Autodesk Fusion 360 part; units mm, degrees
(part 2 of 6)
  constraint perpendicular L499 L505
  constraint perpendicular L506 L507
  constraint perpendicular L505 L506
  constraint perpendicular L478 L508
  constraint parallel L412 L509
  constraint perpendicular L508 L510
  constraint horizontal L511
  constraint vertical L512
  constraint horizontal L513
  constraint vertical L514
  constraint coincident L510 L515.start
  constraint perpendicular L510 L515
  constraint coincident L509 L516.end
  constraint perpendicular L515 L516
  constraint coincident L515.end L516.start
  constraint tangent L509 A143
  constraint tangent L481 A144
  constraint tangent L410 A144
  constraint tangent L407 A145
  constraint tangent L403 A145
  constraint coincident L512.end L513.start
  constraint tangent L480 A147
  constraint tangent L481 A147
  constraint coincident L480 L517.start
  constraint perpendicular L412 L517
  constraint tangent A147 L517
  constraint coincident L481 L518.start
  constraint perpendicular L404 L518
  constraint tangent A147 L518
  constraint coincident L481 L519.start
  constraint perpendicular L481 L519
  constraint tangent A144 L519
  constraint perpendicular L519 L520
  constraint tangent A144 L520
  constraint coincident L410 L520.end
  constraint coincident L477 L521.start
  constraint perpendicular L477 L521
  constraint perpendicular L521 L522
  constraint tangent A145 L521
  constraint tangent A145 L522
  constraint coincident L407 L522.end
  constraint coincident L510 L523.start
  constraint perpendicular L510 L523
  constraint perpendicular L523 L524
  constraint tangent A143 L524
  constraint tangent A143 L523
  constraint coincident L509 L524.end
  constraint coincident L508 L525.start
  constraint perpendicular L508 L525
  constraint coincident L510 L526.end
  constraint perpendicular L510 L526
  constraint tangent A146 L525
  constraint tangent A146 L526
  constraint perpendicular L502 L527
  constraint perpendicular L527 L528
  constraint perpendicular L505 L529
  constraint perpendicular L529 L530
  constraint perpendicular L506 L531
  constraint perpendicular L531 L532
  constraint horizontal L533
  constraint vertical L534
  constraint horizontal L535
  constraint vertical L536
  constraint coincident L495 L534.end
  constraint parallel L504 L535
  constraint coincident L536 A148.centre
  constraint tangent L535 A148
  constraint tangent L535 A149
  constraint tangent L534 A149
  constraint coincident L506 A150.centre
  constraint tangent L507 A150
  constraint coincident L505 A151.centre
  constraint tangent L506 A151
  constraint coincident L501 A152.centre
  constraint tangent L502 A152
  constraint coincident L528.end A153.centre
  constraint coincident L530.end A154.centre
  constraint coincident L532.end A155.centre
  constraint coincident L497.end A156.centre
  constraint coincident L535 L537.start
  constraint perpendicular L535 L537
  constraint coincident L537.end A157.centre
  constraint perpendicular L536 L538
  constraint perpendicular L538 L539
  constraint coincident L539.end A158.centre
  constraint coincident A158 L540.end
  constraint tangent A158 L540
  constraint coincident A158 L541.start
  constraint coincident L503 L541.end
  constraint tangent A158 L541
  constraint perpendicular L503 L541
  constraint coincident A157 L542.end
  constraint tangent A157 L542
  constraint perpendicular L537 L543
  constraint coincident A157 L544.end
  constraint tangent A157 L544
  constraint coincident A156 L545.end
  constraint tangent A156 L545
  constraint perpendicular L497 L546
  constraint coincident A156 L547.end
  constraint tangent A156 L547
  constraint coincident A153 L548.end
  constraint tangent A153 L548
  constraint coincident L506 L549.end
  constraint perpendicular L506 L549
  constraint perpendicular L549 L550
  constraint perpendicular L549 L551
  constraint coincident A155 L552.end
  constraint tangent A155 L552
  constraint coincident A155 L553.end
  constraint tangent A155 L553
  constraint coincident A154 L554.end
  constraint tangent A154 L554
  constraint coincident L505 L555.end
  constraint perpendicular L505 L555
  constraint perpendicular L555 L556
  constraint coincident A154 L557.end
  constraint tangent A154 L557
  constraint coincident L502 L558.end
  constraint perpendicular L502 L558
  constraint perpendicular L558 L559
  constraint coincident A153 L560.end
  constraint tangent A153 L560
  constraint coincident A113.centre L561.start
  constraint coincident L403 L561.end
  constraint perpendicular L477 L561
  constraint coincident L410 L562.start
  constraint vertical L562
  constraint coincident A147.centre L563.end
  constraint parallel L563 L564
  constraint coincident L562.end L564.end
  constraint coincident A60.centre A139.centre
  constraint coincident L562 L565.end
  constraint perpendicular L562 L565
  constraint parallel L565 L566
  constraint perpendicular L566 L567
  constraint perpendicular L566 L568
  constraint coincident L562 L569.start
  constraint coincident L562 L570.end
  constraint perpendicular L520 L574
  constraint horizontal L575
  constraint vertical L576
  constraint horizontal L577
  constraint vertical L578
  constraint perpendicular L575 L579
  constraint coincident L573 L580.start
  constraint perpendicular L579 L581
  constraint perpendicular L573 L580
  constraint parallel L572 L580
  constraint coincident L562 L582.end
  constraint perpendicular L562 L582
  constraint midpoint L49 L583.start
  constraint coincident L580 L583.end
  constraint perpendicular L580 L583
  constraint coincident A51.centre A141.centre
  constraint perpendicular L562 L584
  constraint perpendicular L584 L585
  constraint coincident L507 L586.start
  constraint coincident L507 L586.end
  constraint perpendicular L586 L587
  constraint coincident L564 L588.end
  constraint perpendicular L584 L588
  constraint coincident A125.centre L589.start
  constraint perpendicular L500 L589
  constraint perpendicular L481 L590
  constraint coincident L404 L591.end
  constraint coincident L404 L592.end
  constraint parallel L404 L592
  constraint perpendicular L585 L593
  constraint coincident A57.centre A140.centre
  constraint perpendicular L593 L596
  constraint perpendicular L590 L595
  constraint coincident L562 L597.end
  constraint perpendicular L562 L597
  constraint coincident L562 L599.end
  constraint perpendicular L562 L599
  constraint coincident L404 L600.end
  constraint coincident L481 L601.end
  constraint parallel L590 L600
  constraint parallel L593 L601
  constraint perpendicular L566 L602
  constraint perpendicular L565 L603
  constraint coincident L571 L604.end
  constraint coincident L562 L609.start
  constraint perpendicular L602 L609
  constraint perpendicular L602 L608
  constraint perpendicular L607 L608
  constraint perpendicular L605 L606
  constraint perpendicular L603 L604
  constraint perpendicular L603 L605
  measures "d1" distance of L0.start L0.end
  measures "d2" distance of L12.start L485.end
  measures "d3" distance of L12.start L487.end
  measures "d4" distance of L10.start L489.end
  measures "d5" distance of L10.start L491.end
  measures "d6" distance of L486.end L496.end
  measures "d7" distance of L496.end L497.end
  measures "d8" distance of L490.end L498.end
  measures "d10" distance of L499.start L499.end
  measures "d11" distance of L500.start L500.end
  measures "d12" distance of L502 L503
  measures "d13" distance of L501 L506
  measures "d14" distance of L406 L506
  measures "d15" distance of L403 L404
  measures "d16" distance of L406.start L407.end
  measures "d17" distance of L406.start L508.end
  measures "d18" distance of L508.end L511.end
  measures "d19" distance of L508.end L513.end
  measures "d20" distance of L515.start L515.end
  measures "d22" diameter of A143
  measures "d23" diameter of A144
  measures "d24" diameter of A145
  measures "d25" diameter of A146
  measures "d26" diameter of A147
  measures "d27" distance of L501.end L527.end
  measures "d28" distance of L527.end L528.end
  measures "d29" distance of L505.end L529.end
  measures "d30" distance of L529.end L530.end
  measures "d31" distance of L506.end L531.end
  measures "d32" distance of L531.end L532.end
  measures "d33" distance of L533 L535
  measures "d34" diameter of A148
  measures "d35" diameter of A149
  measures "d36" diameter of A150
  measures "d37" diameter of A151
  measures "d38" diameter of A152
  measures "d39" diameter of A153
  measures "d40" diameter of A154
  measures "d41" diameter of A155
  measures "d42" diameter of A156
  measures "d43" distance of L537.start L537.end
  measures "d44" distance of L534.end L537
  measures "d45" diameter of A157
  measures "d46" distance of L535.end L538.end
  measures "d47" distance of L538.end L539.end
  measures "d48" diameter of A158
  measures "d49" distance of L537.start L543.end
  measures "d50" distance of L496.end L546.end
  measures "d51" distance of L549.end L550.end
  measures "d52" distance of L549.end L551.end
  measures "d53" distance of L555.end L556.end
  measures "d54" distance of L558.end L559.end
  measures "d55" distance of A113.centre L561.end
  measures "d56" distance of A112.centre A113.centre
  measures "d57" distance of L404 L562
  measures "d58" distance of A60.centre L565.end
  measures "d59" distance of A60.centre L566.end
  measures "d60" distance of L566.end L567.end
  measures "d61" distance of L566.end L568.end
  measures "d62" distance of L565.end L570.end
  measures "d63" distance of L565.end L569.start
  measures "d70" angle of L410 L574
  measures "d72" distance of L575.start L575.end
  measures "d73" distance of L575.start L577.end
  measures "d74" distance of A114.centre L575
  measures "d75" distance of A114.centre L576
  measures "d76" distance of L562 L576
  measures "d77" distance of L575.end L579.end
  measures "d80" distance of L583.start L583.end
  measures "d81" distance of A51.centre L562
  measures "d82" distance of A51.centre L584.end
  measures "d84" distance of L586.start L586.end
  measures "d87" distance of A125.centre L589.end
  measures "d88" angle of L562 L598
  measures "d89" angle of L591 L595
  measures "d90" angle of L594 L596
  measures "d91" distance of L590.end A57.centre
  measures "d92" distance of L593.end A57.centre
  measures "d93" distance of A60.centre L603.end
  measures "d94" distance of A60.centre L602.end
sketch "Sketch2" plane through (0, 0, 0) normal (0, 1, 0) x (1, 0, 0)
  line L0 (123.6133, -112.6772) -> (84.9842, -117.4397)
  line L1 (123.6486, -112.6772) -> (118.0197, -90.1409)
  line L2 (121.9175, -105.7465) -> (132.0216, -103.2228)
  line L3 (132.0216, -103.2228) -> (140.1031, -103.2228)
  line L4 (140.1031, -103.2228) -> (142.7339, -103.2228)
  line L5 (142.7339, -107.9103) -> (142.7339, -30.6526)
  line L6 (142.7339, -80.8214) -> (146.7556, -80.8214)
  line L7 (150.7772, -80.8214) -> (146.7556, -80.8214)
  line L8 (149.7839, -80.9328) -> (143.7839, -80.9328)
  circle A0 centre (149.7839, -83.4328) radius 2.5
  line L9 (143.7839, -89.4328) -> (150.9524, -85.6429)
  circle A1 centre (143.7839, -87.4328) radius 2
  line L10 (143.7839, -89.4328) -> (143.7839, -81.4328)
  line L11 (143.7839, -48.2006) -> (143.7839, -81.4328)
  line L12 (150.7772, -76.7997) -> (150.7772, -78.8106)
  line L13 (150.7772, -78.8106) -> (150.7772, -80.8214)
  line L14 (150.7772, -76.7997) -> (150.7772, -74.7889)
  line L15 (150.7772, -72.7781) -> (150.7772, -74.7889)
  line L16 (146.7556, -72.7781) -> (150.7772, -72.7781)
  line L17 (146.7556, -72.7781) -> (142.7339, -72.7781)
  line L18 (144.7094, -48.4919) -> (142.7339, -48.4919)
  line L19 (144.7094, -48.4919) -> (157.6917, -48.4919)
  line L20 (157.6917, -48.4919) -> (161.7839, -48.4919)
  line L21 (157.6917, -40.3375) -> (161.7839, -40.3375)
  line L22 (161.7839, -30.1978) -> (161.7839, -98.4956)
  line L23 (150.7772, -40.3375) -> (157.6917, -40.3375)
  line L24 (150.7772, -37.8883) -> (150.7772, -40.3375)
  line L25 (150.7772, -37.8883) -> (150.7772, -28.4944)
  circle A2 centre (155.7839, -27.151) radius 6
  line L26 (161.7839, -33.151) -> (153.5462, -33.151)
  line L27 (161.7839, -25.5411) -> (161.7839, -103.1522)
  line L28 (161.7839, -25.5411) -> (155.7839, -27.151)
  line L29 (155.7839, -27.151) -> (142.7339, -30.6526)
  line L30 (157.9757, -18.9558) -> (147.6976, -24.893)
  line L31 (143.7839, -15.9328) -> (143.7839, -48.2006)
  circle A3 centre (141.7839, -15.9328) radius 2
  line L32 (27.2428, -15.9328) -> (143.7839, -15.9328)
  line L33 (125.7839, -15.9328) -> (121.994, -8.7643)
  circle A4 centre (119.7839, -9.9328) radius 2.5
  line L34 (113.7839, -15.9328) -> (117.5738, -8.7643)
  line L35 (142.6281, 7.5847) -> (161.7839, -25.5411)
  line L36 (142.6281, 7.5847) -> (103.8578, -14.9931)
  line L37 (9.2428, -14.9931) -> (103.8578, -14.9931)
  circle A5 centre (27.2428, -17.9328) radius 2
  line L38 (27.2428, -15.9328) -> (20.0743, -19.7226)
  circle A6 centre (21.2428, -21.9328) radius 2.5
  line L39 (27.2428, -27.9328) -> (20.0743, -24.1429)
  line L40 (27.2428, -51.1815) -> (27.2428, -15.9328)
  line L41 (27.2428, -81.4328) -> (27.2428, -51.1815)
  line L42 (27.2428, -69.4328) -> (20.0743, -73.2226)
  circle A7 centre (21.2428, -75.4328) radius 2.5
  line L43 (27.2428, -81.4328) -> (20.0743, -77.6429)
  circle A8 centre (29.2428, -81.4328) radius 2
  line L44 (57.5469, -81.4328) -> (27.2428, -81.4328)
  line L45 (51.5469, -81.4328) -> (55.3368, -88.6012)
  circle A9 centre (57.5469, -87.4328) radius 2.5
  line L46 (63.5469, -81.4328) -> (59.7571, -88.6012)
  line L47 (63.5469, -81.6328) -> (63.5469, -117.0186)
  line L48 (63.5469, -81.4328) -> (57.5469, -81.4328)
  line L49 (63.5469, -81.6328) -> (63.5469, -81.4328)
  line L50 (63.5469, -81.4328) -> (63.7469, -81.4328)
  line L51 (63.7469, -81.4328) -> (86.36, -81.4328)
  line L52 (86.56, -81.4328) -> (86.36, -81.4328)
  line L53 (86.56, -81.4328) -> (86.56, -89.4328)
  line L54 (143.7839, -81.4328) -> (86.56, -81.4328)
  line L55 (98.56, -89.4328) -> (94.7701, -96.6012)
  circle A10 centre (92.56, -95.4328) radius 2.5
  line L56 (86.56, -89.4328) -> (90.3499, -96.6012)
  circle A11 centre (88.56, -87.4328) radius 2
  line L57 (86.56, -89.4328) -> (143.7839, -89.4328)
  line L58 (149.7839, -92.4665) -> (149.7839, -106.1494)
  line L59 (161.7839, -92.4665) -> (149.7839, -92.4665)
  circle A12 centre (155.7839, -98.4665) radius 6
  line L60 (161.7839, -103.1522) -> (123.6486, -112.6772)
  line L61 (84.9842, -117.4397) -> (66.9572, -117.4397)
  line L62 (9.2428, -110.3136) -> (66.9572, -117.4397)
  line L63 (21.2428, -99.0089) -> (21.2428, -111.7953)
  line L64 (9.2428, -99.0089) -> (21.2428, -99.0089)
  circle A13 centre (15.2428, -105.0089) radius 6
  line L65 (9.2428, -105.6569) -> (9.2428, -19.6497)
  line L66 (9.2428, -110.3136) -> (9.2428, -14.9931)
  line L67 (142.6281, 7.5847) -> (100.6075, 80.3275)
  line L68 (9.2428, -14.9931) -> (9.2428, 80.3275)
  line L69 (21.2428, 68.3275) -> (21.2428, 80.3275)
  line L70 (9.2428, 68.3275) -> (21.2428, 68.3275)
  circle A14 centre (15.2428, 74.3275) radius 6
  line L71 (91.1443, 80.3275) -> (91.1443, 68.3275)
  line L72 (91.1443, 68.3275) -> (107.5394, 68.3275)
  circle A15 centre (97.1443, 74.3275) radius 6
  line L73 (9.2428, 80.3275) -> (100.6075, 80.3275)
  line L74 (155.7839, -27.151) -> (97.1443, 74.3275)
  line L75 (15.2428, -105.0089) -> (15.2428, 74.3275)
  line L76 (21.2428, -21.9328) -> (15.2428, -21.9328)
  circle A16 centre (15.2428, 26.1974) radius 2.5
  circle A17 centre (126.4641, 23.5882) radius 2.5
  line L77 (15.2428, 68.3275) -> (9.2428, 68.3275)
  line L78 (21.2428, 80.3275) -> (21.2428, 74.3275)
  line L79 (9.2428, 68.3275) -> (9.2428, 80.3275)
  line L80 (21.2428, 80.3275) -> (9.2428, 80.3275)
  line L81 (21.2428, 80.3275) -> (91.1443, 80.3275)
  line L82 (91.1443, 80.3275) -> (91.1443, 74.3275)
  line L83 (107.5394, 68.3275) -> (97.1443, 68.3275)
  arc A18 (91.1443, 74.3275) -> (97.1443, 68.3275) centre (97.1443, 74.3275) ccw
  line L84 (91.1443, 80.3275) -> (100.6075, 80.3275)
  line L85 (100.6075, 80.3275) -> (142.6281, 7.5847)
  line L86 (142.6281, 7.5847) -> (103.8578, -14.9931)
  line L87 (103.8578, -14.9931) -> (9.2428, -14.9931)
  line L88 (9.2428, -110.3136) -> (9.2428, 68.3275)
  line L89 (9.2428, -99.0089) -> (15.2428, -99.0089)
  arc A19 (21.2428, -105.0089) -> (15.2428, -99.0089) centre (15.2428, -105.0089) ccw
  line L90 (21.2428, -105.0089) -> (21.2428, -111.7953)
  line L91 (9.2428, -110.3136) -> (21.2428, -111.7953)
  line L92 (21.2428, -111.7953) -> (66.9572, -117.4397)
  line L93 (66.9572, -117.4397) -> (84.9842, -117.4397)
  line L94 (63.5469, -117.0186) -> (63.5469, -81.4328)
  line L95 (63.5469, -81.4328) -> (59.7571, -88.6012)
  line L96 (63.5469, -81.4328) -> (51.5469, -81.4328)
  line L97 (55.3368, -88.6012) -> (51.5469, -81.4328)
  arc A20 (55.3368, -88.6012) -> (59.7571, -88.6012) centre (57.5469, -87.4328) ccw
  line L98 (51.5469, -81.4328) -> (27.2428, -81.4328)
  arc A21 (27.2428, -81.4328) -> (31.2428, -81.4328) centre (29.2428, -81.4328) ccw
  arc A22 (20.0743, -73.2226) -> (20.0743, -77.6429) centre (21.2428, -75.4328) ccw
  line L99 (27.2428, -81.4328) -> (20.0743, -77.6429)
  line L100 (20.0743, -73.2226) -> (27.2428, -69.4328)
  line L101 (27.2428, -81.4328) -> (27.2428, -69.4328)
  line L102 (27.2428, -69.4328) -> (27.2428, -27.9328)
  line L103 (27.2428, -27.9328) -> (20.0743, -24.1429)
  arc A23 (20.0743, -19.7226) -> (20.0743, -24.1429) centre (21.2428, -21.9328) ccw
  line L104 (20.0743, -19.7226) -> (27.2428, -15.9328)
  arc A24 (27.2428, -15.9328) -> (27.2428, -19.9328) centre (27.2428, -17.9328) ccw
  line L105 (27.2428, -19.9328) -> (27.2428, -27.9328)
  line L106 (27.2428, -15.9328) -> (113.7839, -15.9328)
  line L107 (113.7839, -15.9328) -> (125.7839, -15.9328)
  line L108 (117.5738, -8.7643) -> (113.7839, -15.9328)
  line L109 (121.994, -8.7643) -> (125.7839, -15.9328)
  arc A25 (121.994, -8.7643) -> (117.5738, -8.7643) centre (119.7839, -9.9328) ccw
  arc A26 (143.7839, -15.9328) -> (139.7839, -15.9328) centre (141.7839, -15.9328) ccw
  line L110 (125.7839, -15.9328) -> (139.7839, -15.9328)
  line L111 (139.7839, -15.9328) -> (143.7839, -15.9328)
  line L112 (27.2428, -15.9328) -> (27.2428, -19.9328)
  line L113 (143.7839, -15.9328) -> (143.7839, -80.9328)
  line L114 (143.7839, -80.9328) -> (143.7839, -81.4328)
  line L115 (143.7839, -81.4328) -> (86.56, -81.4328)
  line L116 (86.56, -81.4328) -> (86.56, -89.4328)
  line L117 (63.5469, -81.4328) -> (86.56, -81.4328)
  arc A27 (86.56, -87.4328) -> (88.56, -89.4328) centre (88.56, -87.4328) ccw
  line L118 (86.56, -89.4328) -> (90.3499, -96.6012)
  line L119 (94.7701, -96.6012) -> (98.56, -89.4328)
  line L120 (88.56, -89.4328) -> (98.56, -89.4328)
  arc A28 (90.3499, -96.6012) -> (94.7701, -96.6012) centre (92.56, -95.4328) ccw
  line L121 (98.56, -89.4328) -> (143.7839, -89.4328)
  line L122 (143.7839, -89.4328) -> (143.7839, -85.4328)
  line L123 (143.7839, -81.4328) -> (143.7839, -85.4328)
  line L124 (143.7839, -89.4328) -> (150.9524, -85.6429)
  line L125 (143.7839, -80.9328) -> (149.7839, -80.9328)
  arc A29 (143.7839, -89.4328) -> (143.7839, -85.4328) centre (143.7839, -87.4328) ccw
  arc A30 (150.9524, -85.6429) -> (149.7839, -80.9328) centre (149.7839, -83.4328) ccw
  line L126 (142.6281, 7.5847) -> (161.7839, -25.5411)
  arc A31 (152.7827, -21.9556) -> (155.7839, -33.151) centre (155.7839, -27.151) ccw
  line L127 (155.7839, -33.151) -> (161.7839, -33.151)
  line L128 (157.9757, -18.9558) -> (152.7827, -21.9556)
  line L129 (161.7839, -25.5411) -> (161.7839, -33.151)
  line L130 (161.7839, -33.151) -> (161.7839, -40.3375)
  line L131 (161.7839, -40.3375) -> (161.7839, -48.4919)
  line L132 (123.6486, -112.6772) -> (84.9842, -117.4397)
  line L133 (123.6486, -112.6772) -> (121.9175, -105.7465)
  line L134 (121.9175, -105.7465) -> (132.0216, -103.2228)
  line L135 (132.0216, -103.2228) -> (140.1031, -103.2228)
  line L136 (140.1031, -103.2228) -> (142.7339, -103.2228)
  line L137 (123.6486, -112.6772) -> (142.7339, -107.9103)
  line L138 (142.7339, -107.9103) -> (149.7839, -106.1494)
  line L139 (149.7839, -106.1494) -> (161.7839, -103.1522)
  line L140 (142.7339, -103.2228) -> (142.7339, -80.8214)
  line L141 (142.7339, -80.8214) -> (150.7772, -80.8214)
  line L142 (150.7772, -80.8214) -> (150.7772, -72.7781)
  line L143 (150.7772, -72.7781) -> (142.7339, -72.7781)
  arc A32 (155.7839, -92.4665) -> (149.7839, -98.4665) centre (155.7839, -98.4665) ccw
  line L144 (149.7839, -98.4665) -> (149.7839, -106.1494)
  line L145 (155.7839, -92.4665) -> (161.7839, -92.4665)
  line L146 (161.7839, -103.1522) -> (161.7839, -92.4665)
  line L147 (161.7839, -92.4665) -> (161.7839, -48.4919)
  line L148 (161.7839, -48.4919) -> (142.7339, -48.4919)
  line L149 (161.7839, -40.3375) -> (150.7772, -40.3375)
  line L150 (150.7772, -40.3375) -> (150.7772, -28.4944)
  line L151 (150.7772, -28.4944) -> (161.7839, -25.5411)
  line L152 (86.56, -89.4328) -> (86.56, -117.2454)
  line L153 (142.7339, -72.7781) -> (142.7339, -48.4919)
  line L154 (161.7839, -48.4919) -> (157.6917, -44.4147)
  line L155 (150.7772, -40.3375) -> (146.7556, -37.8883)
  line L156 (146.7556, -76.7997) -> (150.7772, -72.7781)
  arc A33 (15.2428, 68.3275) -> (21.2428, 74.3275) centre (15.2428, 74.3275) ccw
  arc A34 (146.7556, -80.8214) -> (146.7556, -72.7781) centre (146.7556, -76.7997) ccw
  line L157 (146.7556, -76.7997) -> (146.7556, -72.7781)
  line L158 (146.7556, -72.7781) -> (146.7556, -68.7564)
  arc A35 (142.7339, -68.7564) -> (146.7556, -72.7781) centre (146.7556, -68.7564) ccw
  line L159 (146.7556, -76.7997) -> (146.7556, -84.843)
  arc A36 (146.7556, -80.8214) -> (142.7339, -84.843) centre (146.7556, -84.843) ccw
  arc A37 (157.6917, -48.4919) -> (157.6917, -40.3375) centre (157.6917, -44.4147) ccw
  line L160 (150.7772, -40.3375) -> (154.8544, -36.2603)
  arc A38 (150.7772, -36.2632) -> (154.8573, -40.3375) centre (154.8544, -36.2603) ccw
  line L161 (154.8544, -36.2603) -> (154.8544, -27.4004)
  line L162 (153.7978, -27.6839) -> (154.8544, -31.6219)
  arc A39 (153.7978, -27.6839) -> (150.7772, -31.6219) centre (154.8544, -31.6219) ccw
  line L163 (142.7339, -52.5692) -> (146.8111, -52.5692)
  line L164 (146.8111, -52.5692) -> (146.8111, -48.4919)
  arc A40 (146.8111, -48.4919) -> (142.7339, -52.5692) centre (146.8111, -52.5692) ccw
  line L165 (142.7339, -103.2228) -> (138.7122, -99.2011)
  arc A41 (138.7122, -103.2228) -> (142.7339, -99.2011) centre (138.7122, -99.2011) ccw
  line L166 (121.9175, -105.7465) -> (126.7939, -108.6737)
  line L167 (126.7939, -108.6737) -> (125.8193, -104.7719)
  arc A42 (125.8193, -104.7719) -> (122.8921, -109.6483) centre (126.7939, -108.6737) ccw
  line L168 (132.0216, -103.2228) -> (132.5125, -107.2144)
  arc A43 (132.5125, -103.2228) -> (131.5453, -103.3417) centre (132.5125, -107.2144) ccw
  line L169 (15.2428, 74.3275) -> (97.1443, 74.3275)
  circle A44 centre (56.1936, 74.3275) radius 2.5
  arc A45 (15.2428, 80.3275) -> (9.2428, 74.3275) centre (15.2428, 74.3275) ccw
  arc A46 (102.3398, 77.3287) -> (97.1443, 80.3275) centre (97.1443, 74.3275) ccw
  point P0 (146.7556, -76.7997)
  point P1 (157.6917, -44.4147)
  point P2 (146.7556, -37.8883)
  dimension "d95" = 5
  dimension "d96" = 5
  dimension "d97" = 58.6014
  dimension "d98" = 58.6014
  dimension "d99" = 48.1301
  dimension "d100" = 48.1301
  dimension "d101" = 4.0217
  dimension "d102" = 4.0217
  dimension "d103" = 8.0433
  dimension "d104" = 4.0772
  dimension "d105" = 4.0922
  dimension "d106" = 4.0772
  dimension "d107" = 4.0772
  dimension "d108" = 4.0772
  dimension "d109" = 4.0772
  dimension "d110" = 4.0772
  dimension "d111" = 4.0217
  dimension "d112" = 4.0217
  dimension "d113" = 4.0217
  dimension "d114" = 4.0217
  dimension "d115" = 82.988
  dimension "d116" = 82.988
  dimension "d117" = 4.0217
  dimension "d118" = 5
  constraint coincident A2.centre L28.end
  constraint coincident A15.centre L74.end
  constraint coincident A13.centre L75.start
  constraint coincident A14.centre L75.end
  constraint coincident A6.centre L76.start
  constraint coincident L75 L76.end
  constraint perpendicular L75 L76
  constraint coincident L75 A16.centre
  constraint coincident L74 A17.centre
  constraint midpoint L70 L77.start
  constraint coincident L70.start L77.end
  constraint coincident L69.end L78.start
  constraint midpoint L69 L78.end
  constraint coincident L68.end L73.start
  constraint coincident L71.start L81.end
  constraint midpoint L71 L82.end
  constraint coincident L72.end L83.start
  constraint coincident A15 L83.end
  constraint coincident L72 L83.end
  constraint coincident L67.end L73.end
  constraint coincident L35.start L36.start
  constraint coincident L36.end L37.end
  constraint coincident L37.start L66.end
  constraint coincident L62.start L66.start
  constraint coincident L64.start L89.start
  constraint midpoint L64 L89.end
  constraint coincident L63.end L90.end
  constraint tangent A13 L90
  constraint coincident L61.end L62.end
  constraint coincident L0.end L61.start
  constraint coincident L47.end L94.start
  constraint coincident L46.start L48.start
  constraint coincident L46.end L95.end
  constraint coincident L45.start L96.end
  constraint coincident L45.end L97.start
  constraint coincident A9.centre A20.centre
  constraint coincident L41.start L43.start
  constraint coincident A8 A21.end
  constraint coincident L44 A21.end
  constraint coincident A8.centre A21.centre
  constraint coincident L43.end A22.end
  constraint coincident L42.end A22.start
  constraint coincident A7.centre A22.centre
  constraint coincident L42.start L100.end
  constraint coincident L39.start L102.end
  constraint coincident L39.end L103.end
  constraint coincident L38.end A23.start
  constraint coincident L32.start L38.start
  constraint coincident L40 A24.end
  constraint coincident A5 A24.end
  constraint coincident A5.centre A24.centre
  constraint coincident L34.start L106.end
  constraint coincident L33.start L107.end
  constraint coincident L34.end L108.start
  constraint coincident L33.end L109.start
  constraint coincident A4.centre A25.centre
  constraint coincident L31.start L32.end
  constraint coincident A3 A26.end
  constraint coincident L32 A26.end
  constraint coincident A3.centre A26.centre
  constraint coincident L8.end L113.end
  constraint coincident L10.end L11.end
  constraint coincident L52.start L53.start
  constraint coincident L53.end L56.start
  constraint coincident L57 A27.end
  constraint coincident A11 A27.start
  constraint coincident A11.centre A27.centre
  constraint coincident L56.end L118.end
  constraint coincident L55.end L119.start
  constraint coincident L55.start L119.end
  constraint coincident A10.centre A28.centre
  constraint coincident L9.start L10.start
  constraint midpoint L10 L122.end
  constraint coincident L9.end L124.end
  constraint coincident L8.start L125.end
  constraint coincident A1.centre A29.centre
  constraint coincident A0.centre A30.centre
  constraint coincident L27.start L28.start
  constraint coincident L26 A31.end
  constraint coincident A2 A31.start
  constraint coincident L26.start L127.end
  constraint coincident L30.start L128.start
  constraint tangent A2 L128
  constraint coincident L21.end L130.end
  constraint coincident L20.end L131.end
  constraint coincident L1.start L60.end
  constraint coincident L2.start L133.end
  constraint coincident L2.end L3.start
  constraint coincident L3.end L4.start
  constraint coincident L4.end L136.end
  constraint coincident L5.start L137.end
  constraint coincident L58.end L138.end
  constraint coincident L27.end L60.start
  constraint coincident L6.start L140.end
  constraint coincident L7.start L13.end
  constraint coincident L15.start L16.end
  constraint coincident L17.end L143.end
  constraint midpoint L59 A32.start
  constraint coincident A12.centre A32.centre
  constraint tangent A32 L144
  constraint coincident L59.start L145.end
  constraint coincident L18.end L148.end
  constraint coincident L23.start L24.end
  constraint coincident L25.end L150.end
  constraint coincident L0 L152.end
  constraint parallel L150 L152
  constraint coincident P1 L154.end
  constraint coincident P2 L155.end
  constraint coincident P0 L156.start
  constraint coincident L16.start L17.start
  constraint coincident L6.end L7.end
  constraint perpendicular L143 L158
  constraint coincident L5 A35.start
  constraint coincident L158.end A35.centre
  constraint perpendicular L125 L159
  constraint coincident L5 A36.end
  constraint coincident L159.end A36.centre
  constraint coincident L21.start L23.end
  constraint coincident L19.end L20.start
  constraint coincident L23 A38.end
  constraint coincident L150 A38.start
  constraint coincident L160.end A38.centre
  constraint coincident L151 L161.end
  constraint parallel L25 L161
  constraint coincident L151 L162.start
  constraint coincident L161 L162.end
  constraint perpendicular L29 L162
  constraint coincident L25 A39.end
  constraint coincident L162.end A39.centre
  constraint coincident L153 L163.start
  constraint perpendicular L153 L163
  constraint coincident L148 L164.end
  constraint perpendicular L163 L164
  constraint coincident L5 A41.end
  constraint coincident L135 A41.start
  constraint coincident L165.end A41.centre
  constraint coincident L134 L167.end
  constraint perpendicular L134 L167
  constraint coincident L1 A42.end
  constraint coincident L166.end L167.start
  constraint coincident L134 A43.end
  constraint coincident L135 A43.start
  constraint coincident L168.end A43.centre
  constraint parallel L81 L169
  constraint midpoint L169 A44.centre
  constraint coincident L79 A45.end
  constraint midpoint L80 A45.start
  constraint coincident L67 A46.start
  constraint coincident L84 A46.end
  constraint coincident A15 A46.end
  measures "d95" diameter of A16
  measures "d96" diameter of A17
  measures "d97" distance of A15.centre A17.centre
  measures "d98" distance of A2.centre A17.centre
  measures "d99" distance of L76 A16.centre
  measures "d100" distance of A14.centre A16.centre
  measures "d101" distance of L16.start L158.end
  measures "d102" distance of P0 L16.start
  measures "d103" distance of P0 L159.end
  measures "d104" distance of P1 L19.end
  measures "d105" distance of L131 P1
  measures "d106" distance of L149 L160.end
  measures "d107" distance of L150 L160.end
  measures "d108" distance of L162.start L162.end
  measures "d109" distance of L163.end L164.end
  measures "d110" distance of L163.start L163.end
  measures "d111" distance of L4 L165.end
  measures "d112" distance of L5 L165.end
  measures "d113" distance of L2 L166.end
  measures "d114" distance of L1 L166.end
  measures "d115" angle of L2 L168
  measures "d116" angle of L3 L168
  measures "d117" distance of L2.end L168.end
  measures "d118" diameter of A44
sketch "battery plate" plane through (0, 0, 0) normal (0, 1, 0) x (1, 0, 0)
  line L0 (20.0743, -19.7226) -> (27.2428, -15.9328)
  arc A0 (20.0743, -19.7226) -> (20.0743, -24.1429) centre (21.2428, -21.9328) ccw
  line L1 (27.2428, -27.9328) -> (20.0743, -24.1429)
  line L2 (27.2428, -69.4328) -> (27.2428, -27.9328)
  line L3 (27.2428, -15.9328) -> (113.7839, -15.9328)
  line L4 (117.5738, -8.7643) -> (113.7839, -15.9328)
  arc A1 (121.994, -8.7643) -> (117.5738, -8.7643) centre (119.7839, -9.9328) ccw
  line L5 (121.994, -8.7643) -> (125.7839, -15.9328)
  line L6 (125.7839, -15.9328) -> (139.7839, -15.9328)
  line L7 (139.7839, -15.9328) -> (143.7839, -15.9328)
  line L8 (143.7839, -15.9328) -> (143.7839, -80.9328)
  line L9 (143.7839, -80.9328) -> (149.7839, -80.9328)
  arc A2 (150.9524, -85.6429) -> (149.7839, -80.9328) centre (149.7839, -83.4328) ccw
  line L10 (143.7839, -89.4328) -> (150.9524, -85.6429)
  line L11 (98.56, -89.4328) -> (143.7839, -89.4328)
  line L12 (94.7701, -96.6012) -> (98.56, -89.4328)
  arc A3 (90.3499, -96.6012) -> (94.7701, -96.6012) centre (92.56, -95.4328) ccw
  line L13 (86.56, -89.4328) -> (90.3499, -96.6012)
  line L14 (86.56, -81.4328) -> (86.56, -89.4328)
  line L15 (63.5469, -81.4328) -> (86.56, -81.4328)
  line L16 (63.5469, -81.4328) -> (59.7571, -88.6012)
  arc A4 (55.3368, -88.6012) -> (59.7571, -88.6012) centre (57.5469, -87.4328) ccw
  line L17 (55.3368, -88.6012) -> (51.5469, -81.4328)
  line L18 (51.5469, -81.4328) -> (27.2428, -81.4328)
  line L19 (27.2428, -81.4328) -> (20.0743, -77.6429)
  arc A5 (20.0743, -73.2226) -> (20.0743, -77.6429) centre (21.2428, -75.4328) ccw
  line L20 (20.0743, -73.2226) -> (27.2428, -69.4328)
  circle A6 centre (21.2428, -21.9328) radius 1.6
  circle A7 centre (21.2428, -21.9328) radius 1.6
  circle A8 centre (21.2428, -75.4328) radius 1.6
  circle A9 centre (57.5469, -87.4328) radius 1.6
  circle A10 centre (92.56, -95.4328) radius 1.6
  circle A11 centre (149.7839, -83.4328) radius 1.6
  circle A12 centre (119.7839, -9.9328) radius 1.6
  point P0 (21.2428, -21.9328)
  point P1 (119.7839, -9.9328)
  point P2 (149.7839, -83.4328)
  point P3 (92.56, -95.4328)
  point P4 (57.5469, -87.4328)
  point P5 (21.2428, -75.4328)
  dimension "d119" = 3.2
  dimension "d120" = 3.2
  dimension "d121" = 3.2
  dimension "d122" = 3.2
  dimension "d123" = 3.2
  dimension "d124" = 3.2
  dimension "d125" = 3.2
  constraint concentric A0 A6
  constraint coincident P5 A5.centre
  constraint coincident P4 A4.centre
  constraint concentric A3 A10
  constraint coincident P2 A2.centre
  constraint coincident P1 A1.centre
  measures "d119" diameter of A6
  measures "d120" diameter of A7
  measures "d121" diameter of A8
  measures "d122" diameter of A9
  measures "d123" diameter of A10
  measures "d124" diameter of A11
  measures "d125" diameter of A12
sketch "underplate" plane through (0, 0, 0) normal (0, 1, 0) x (1, 0, 0)
  line L0 (21.2428, -105.0089) -> (21.2428, -111.7953)
  arc A0 (21.2428, -105.0089) -> (15.2428, -99.0089) centre (15.2428, -105.0089) ccw
  line L1 (9.2428, -99.0089) -> (15.2428, -99.0089)
  line L2 (15.2428, 68.3275) -> (9.2428, 68.3275)
  arc A1 (15.2428, 68.3275) -> (21.2428, 74.3275) centre (15.2428, 74.3275) ccw
  line L3 (21.2428, 80.3275) -> (21.2428, 74.3275)
  line L4 (21.2428, 80.3275) -> (91.1443, 80.3275)
  line L5 (91.1443, 80.3275) -> (91.1443, 74.3275)
  arc A2 (91.1443, 74.3275) -> (97.1443, 68.3275) centre (97.1443, 74.3275) ccw
  line L6 (107.5394, 68.3275) -> (97.1443, 68.3275)
  line L7 (21.2428, -111.7953) -> (66.9572, -117.4397)
  line L8 (66.9572, -117.4397) -> (84.9842, -117.4397)
  line L9 (123.6486, -112.6772) -> (84.9842, -117.4397)
  line L10 (123.6486, -112.6772) -> (142.7339, -107.9103)
  line L11 (142.7339, -107.9103) -> (149.7839, -106.1494)
  line L12 (149.7839, -98.4665) -> (149.7839, -106.1494)
  arc A3 (155.7839, -92.4665) -> (149.7839, -98.4665) centre (155.7839, -98.4665) ccw
  line L13 (155.7839, -92.4665) -> (161.7839, -92.4665)
  line L14 (161.7839, -92.4665) -> (161.7839, -48.4919)
  line L15 (161.7839, -40.3375) -> (161.7839, -48.4919)
  line L16 (161.7839, -33.151) -> (161.7839, -40.3375)
  line L17 (155.7839, -33.151) -> (161.7839, -33.151)
  arc A4 (152.7827, -21.9556) -> (155.7839, -33.151) centre (155.7839, -27.151) ccw
  line L18 (157.9757, -18.9558) -> (152.7827, -21.9556)
  line L19 (27.2428, -69.4328) -> (27.2428, -27.9328)
  line L20 (27.2428, -81.4328) -> (27.2428, -69.4328)
  arc A5 (27.2428, -81.4328) -> (31.2428, -81.4328) centre (29.2428, -81.4328) ccw
  line L21 (63.5469, -81.4328) -> (51.5469, -81.4328)
  line L22 (63.5469, -81.4328) -> (86.56, -81.4328)
  arc A6 (86.56, -87.4328) -> (88.56, -89.4328) centre (88.56, -87.4328) ccw
  line L23 (88.56, -89.4328) -> (98.56, -89.4328)
  line L24 (98.56, -89.4328) -> (143.7839, -89.4328)
  arc A7 (143.7839, -89.4328) -> (143.7839, -85.4328) centre (143.7839, -87.4328) ccw
  line L25 (143.7839, -81.4328) -> (143.7839, -85.4328)
  line L26 (143.7839, -80.9328) -> (143.7839, -81.4328)
  line L27 (143.7839, -15.9328) -> (143.7839, -80.9328)
  arc A8 (143.7839, -15.9328) -> (139.7839, -15.9328) centre (141.7839, -15.9328) ccw
  line L28 (125.7839, -15.9328) -> (139.7839, -15.9328)
  line L29 (113.7839, -15.9328) -> (125.7839, -15.9328)
  line L30 (27.2428, -15.9328) -> (113.7839, -15.9328)
  arc A9 (27.2428, -15.9328) -> (27.2428, -19.9328) centre (27.2428, -17.9328) ccw
  line L31 (27.2428, -19.9328) -> (27.2428, -27.9328)
  line L32 (9.2428, -99.0089) -> (9.2428, 68.3275)
  line L33 (107.5394, 68.3275) -> (157.9757, -18.9558)
  line L34 (86.56, -87.4328) -> (86.56, -81.4328)
  line L35 (31.2428, -81.4328) -> (51.5469, -81.4328)
  point P0 (97.1443, 74.3275)
  point P1 (15.2428, 74.3275)
  point P2 (15.2428, -105.0089)
  point P3 (155.7839, -98.4665)
  point P4 (155.7839, -27.151)
  point P5 (149.7839, -83.4328)
  point P6 (146.7556, -76.7997)
  point P7 (92.56, -95.4328)
  point P8 (57.5469, -87.4328)
  point P9 (21.2428, -75.4328)
  point P10 (21.2428, -21.9328)
  point P11 (119.7839, -9.9328)
  point P12 (146.7556, -37.8883)
  point P13 (157.6917, -44.4147)
  point P14 (15.2428, 26.1974)
  point P15 (126.4641, 23.5882)
  constraint coincident L1.start L32.start
  constraint coincident L2.end L32.end
  constraint coincident L6.start L33.start
  constraint coincident L18.start L33.end
  constraint coincident A6.start L34.start
  constraint coincident L22.end L34.end
  constraint coincident A5.end L35.start
  constraint coincident L21.end L35.end
sketch "baseplate" plane through (0, 0, 0) normal (0, 1, 0) x (1, 0, 0)
  line L0 (9.2428, -110.3136) -> (9.2428, 68.3275)
  line L1 (9.2428, -110.3136) -> (21.2428, -111.7953)
  line L2 (63.5469, -117.0186) -> (63.5469, -81.4328)
  line L3 (86.56, -89.4328) -> (86.56, -117.2454)
  line L4 (88.56, -89.4328) -> (98.56, -89.4328)
  line L5 (98.56, -89.4328) -> (143.7839, -89.4328)
  arc A0 (143.7839, -89.4328) -> (143.7839, -85.4328) centre (143.7839, -87.4328) ccw
  line L6 (143.7839, -81.4328) -> (143.7839, -85.4328)
  line L7 (143.7839, -80.9328) -> (143.7839, -81.4328)
  line L8 (143.7839, -15.9328) -> (143.7839, -80.9328)
  arc A1 (143.7839, -15.9328) -> (139.7839, -15.9328) centre (141.7839, -15.9328) ccw
  line L9 (125.7839, -15.9328) -> (139.7839, -15.9328)
  line L10 (113.7839, -15.9328) -> (125.7839, -15.9328)
  line L11 (27.2428, -15.9328) -> (113.7839, -15.9328)
  arc A2 (27.2428, -15.9328) -> (27.2428, -19.9328) centre (27.2428, -17.9328) ccw
  line L12 (27.2428, -19.9328) -> (27.2428, -27.9328)
  line L13 (27.2428, -69.4328) -> (27.2428, -27.9328)
  line L14 (27.2428, -81.4328) -> (27.2428, -69.4328)
  arc A3 (27.2428, -81.4328) -> (31.2428, -81.4328) centre (29.2428, -81.4328) ccw
  line L15 (63.5469, -81.4328) -> (51.5469, -81.4328)
  line L16 (123.6486, -112.6772) -> (142.7339, -107.9103)
  line L17 (142.7339, -107.9103) -> (149.7839, -106.1494)
  line L18 (149.7839, -106.1494) -> (161.7839, -103.1522)
  line L19 (161.7839, -103.1522) -> (161.7839, -92.4665)
  line L20 (161.7839, -92.4665) -> (161.7839, -48.4919)
  line L21 (161.7839, -40.3375) -> (161.7839, -48.4919)
  line L22 (161.7839, -33.151) -> (161.7839, -40.3375)
  line L23 (161.7839, -25.5411) -> (161.7839, -33.151)
  line L24 (142.6281, 7.5847) -> (161.7839, -25.5411)
  line L25 (21.2428, 80.3275) -> (91.1443, 80.3275)
  line L26 (88.56, -89.4328) -> (86.56, -89.4328)
  line L27 (21.2428, -111.7953) -> (63.5469, -117.0186)
  line L28 (51.5469, -81.4328) -> (31.2428, -81.4328)
  line L29 (86.56, -117.2454) -> (123.6486, -112.6772)
  arc A4 (15.2428, 80.3275) -> (9.2428, 74.3275) centre (15.2428, 74.3275) ccw
  arc A5 (102.3398, 77.3287) -> (97.1443, 80.3275) centre (97.1443, 74.3275) ccw
  line L30 (9.2428, 68.3275) -> (9.2428, 74.3275)
  line L31 (21.2428, 80.3275) -> (15.2428, 80.3275)
  line L32 (91.1443, 80.3275) -> (97.1443, 80.3275)
  line L33 (142.6281, 7.5847) -> (102.3398, 77.3287)
  circle A6 centre (15.2428, 74.3275) radius 2.5
  circle A7 centre (97.1443, 74.3275) radius 2.5
  circle A8 centre (21.2428, -21.9328) radius 2.5
  circle A9 centre (155.7839, -27.151) radius 2.5
  circle A10 centre (15.2428, -105.0089) radius 2.5
  circle A11 centre (92.56, -95.4328) radius 2.5
  circle A12 centre (57.5469, -87.4328) radius 2.5
  circle A13 centre (155.7839, -98.4665) radius 2.5
  circle A14 centre (21.2428, -75.4328) radius 2.5
  circle A15 centre (149.7839, -83.4328) radius 2.5
  circle A16 centre (28.3281, -91.2283) radius 1.6
  circle A17 centre (123.5781, -102.5878) radius 1.6
  circle A18 centre (146.7556, -76.7997) radius 1.6
  circle A19 centre (157.6917, -44.4147) radius 1.6
  circle A20 centre (18.8031, -34.0783) radius 1.6
  circle A21 centre (119.7839, -9.9328) radius 2.5
  circle A22 centre (130.9158, -10.2658) radius 1.6
  circle A23 centre (146.7556, -37.8883) radius 1.6
  point P0 (15.2428, -105.0089)
  point P1 (57.5469, -87.4328)
  point P2 (21.2428, -75.4328)
  point P3 (21.2428, -21.9328)
  point P4 (119.7839, -9.9328)
  point P5 (146.7556, -37.8883)
  point P6 (157.6917, -44.4147)
  point P7 (146.7556, -76.7997)
  point P8 (92.56, -95.4328)
  point P9 (123.5781, -102.5878)
  point P10 (28.3281, -91.2283)
  point P11 (130.9158, -10.2658)
  point P12 (56.1936, 74.3275)
  point P13 (15.2428, 26.1974)
  point P14 (126.4641, 23.5882)
  point P15 (18.8031, -34.0783)
  point P16 (155.7839, -27.151)
  point P17 (155.7839, -98.4665)
  point P18 (149.7839, -83.4328)
  dimension "d308" = 5
  dimension "d310" = 5
  dimension "d313" = 5
  dimension "d314" = 5
  dimension "d315" = 5
  dimension "d316" = 5
  dimension "d317" = 5
  dimension "d318" = 5
  dimension "d319" = 5
  dimension "d320" = 5
  dimension "d341" = 3.2
  dimension "d342" = 3.2
  dimension "d343" = 3.2
  dimension "d344" = 3.2
  dimension "d345" = 3.2
  dimension "d346" = 5
  dimension "d347" = 3.2
  dimension "d348" = 3.2
  constraint coincident L4.start L26.start
  constraint coincident L3.start L26.end
  constraint coincident L1.end L27.start
  constraint coincident L2.start L27.end
  constraint coincident L15.end L28.start
  constraint coincident A3.end L28.end
  constraint coincident L3.end L29.start
  constraint coincident L16.start L29.end
  constraint coincident L0.end L30.start
  constraint coincident A4.end L30.end
  constraint coincident L25.start L31.start
  constraint coincident A4.start L31.end
  constraint coincident L25.end L32.start
  constraint coincident A5.end L32.end
  constraint coincident L24.start L33.start
  constraint coincident A5.start L33.end
  constraint concentric A4 A6
  constraint concentric A5 A7
  constraint coincident P3 A8.centre
  constraint coincident P16 A9.centre
  constraint coincident P0 A10.centre
  constraint coincident P8 A11.centre
  constraint coincident P1 A12.centre
  constraint coincident P17 A13.centre
  constraint coincident P2 A14.centre
  constraint coincident P18 A15.centre
  constraint coincident P10 A16.centre
  constraint coincident P9 A17.centre
  constraint coincident P7 A18.centre
  constraint coincident P6 A19.centre
  constraint coincident P15 A20.centre
  constraint coincident P4 A21.centre
  constraint coincident P11 A22.centre
  constraint coincident P5 A23.centre
  measures "d308" diameter of A6
  measures "d310" diameter of A7
  measures "d313" diameter of A8
  measures "d314" diameter of A9
  measures "d315" diameter of A10
  measures "d316" diameter of A11
  measures "d317" diameter of A12
  measures "d318" diameter of A13
  measures "d319" diameter of A14
  measures "d320" diameter of A15
  measures "d341" diameter of A16
  measures "d342" diameter of A17
  measures "d343" diameter of A18
  measures "d344" diameter of A19
  measures "d345" diameter of A20
  measures "d346" diameter of A21
  measures "d347" diameter of A22
  measures "d348" diameter of A23
sketch "PCB" plane through (0, 0, 0) normal (0, 1, 0) x (1, 0, 0)
  line L0 (21.2428, -111.7953) -> (66.9572, -117.4397)
  line L1 (66.9572, -117.4397) -> (84.9842, -117.4397)
  line L2 (123.6486, -112.6772) -> (84.9842, -117.4397)
  line L3 (123.6486, -112.6772) -> (142.7339, -107.9103)
  line L4 (142.7339, -107.9103) -> (149.7839, -106.1494)
  line L5 (149.7839, -106.1494) -> (161.7839, -103.1522)
  line L6 (161.7839, -103.1522) -> (161.7839, -92.4665)
  line L7 (161.7839, -92.4665) -> (161.7839, -48.4919)
  line L8 (161.7839, -40.3375) -> (161.7839, -48.4919)
  line L9 (161.7839, -33.151) -> (161.7839, -40.3375)
  line L10 (161.7839, -25.5411) -> (161.7839, -33.151)
  line L11 (142.6281, 7.5847) -> (161.7839, -25.5411)
  line L12 (142.6281, 7.5847) -> (103.8578, -14.9931)
  line L13 (103.8578, -14.9931) -> (9.2428, -14.9931)
  line L14 (9.2428, -110.3136) -> (21.2428, -111.7953)
  line L15 (9.2428, -14.9931) -> (9.2428, -110.3136)
  constraint coincident L13.end L15.start
  constraint coincident L14.start L15.end
sketch "wrist rest" plane through (0, 0, 0) normal (0, 1, 0) x (1, 0, 0)
  line L0 (103.8578, -14.9931) -> (9.2428, -14.9931)
  line L1 (142.6281, 7.5847) -> (103.8578, -14.9931)
  arc A0 (102.3398, 77.3287) -> (97.1443, 80.3275) centre (97.1443, 74.3275) ccw
  arc A1 (15.2428, 80.3275) -> (9.2428, 74.3275) centre (15.2428, 74.3275) ccw
  line L2 (9.2428, -14.9931) -> (9.2428, 74.3275)
  line L3 (15.2428, 80.3275) -> (97.1443, 80.3275)
  line L4 (142.6281, 7.5847) -> (102.3398, 77.3287)
  constraint coincident L0.end L2.start
  constraint coincident A1.end L2.end
  constraint coincident A1.start L3.start
  constraint coincident A0.end L3.end
  constraint coincident L1.start L4.start
  constraint coincident A0.start L4.end